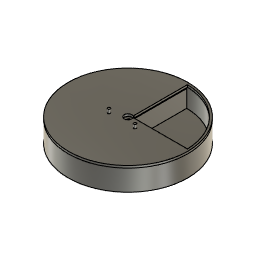
candy-dispenser (Autodesk Fusion 360 design; units mm, degrees)
Autodesk Fusion 360 part; units mm, degrees
note: some values were not read from the file. Set by a fixed rule: which sketch regions a step uses.
sketch "Floor" plane through (0, 0, 0) normal (0, 0, 1) x (1, 0, 0) in component "Container"
  circle A0 centre (0, 0) radius 80
  dimension "d25" = 160
  constraint coincident A0.centre origin
  measures "d25" diameter of A0
extrude "Extrude1" add sketch "Floor" along normal blind 3 makes body 1 in component "Container"
sketch "Walls" plane through (0, 0, 3) normal (0, 0, 1) x (-1, 0, 0) in component "Container"
  circle A0 centre (0, 0) radius 80
  circle A1 centre (0, 0) radius 77.2
  dimension "d28" = -2.8
extrude "Extrude2" add sketch "Walls" along normal blind 25 bodies 1 in component "Container"
sketch "Swiper" plane through (0, 0, 3) normal (0, 0, 1) x (-1, 0, 0) in component "Container"
  circle A0 centre (0, 0) radius 77.2
  line L0 (-80, 2.5) -> (80, 2.5)
  line L1 (80, 2.5) -> (80, -2.5)
  line L2 (80, -2.5) -> (-80, -2.5)
  line L3 (-80, -2.5) -> (-80, 2.5)
  line L4 (-80, 2.5) -> (80, -2.5) construction
  line L5 (80, 2.5) -> (-80, -2.5) construction
  line L6 (-2.5, 80) -> (2.5, 80)
  line L7 (2.5, 80) -> (2.5, -80)
  line L8 (2.5, -80) -> (-2.5, -80)
  line L9 (-2.5, -80) -> (-2.5, 80)
  line L10 (-2.5, 80) -> (2.5, -80) construction
  line L11 (2.5, 80) -> (-2.5, -80) construction
  circle A1 centre (0, 0) radius 6
  circle A2 centre (0, 0) radius 76.2
  dimension "d31" = 160
  dimension "d32" = 5
  dimension "d33" = 5
  dimension "d34" = 160
  dimension "d35" = 12
  dimension "d41" = -1
  constraint horizontal L0
  constraint perpendicular L0 L1
  constraint parallel L0 L2
  constraint parallel L1 L3
  constraint coincident L4 A0.centre
  constraint coincident L5 A0.centre
  constraint coincident A0.centre A1.centre
  constraint horizontal L6
  constraint perpendicular L6 L7
  constraint parallel L6 L8
  constraint parallel L7 L9
  constraint coincident L10 A0.centre
  constraint coincident L11 A0.centre
  measures "d31" distance of L1.end L2.end
  measures "d32" distance of L0.end L1.end
  measures "d33" distance of L7.end L8.end
  measures "d34" distance of L6.end L7.end
  measures "d35" diameter of A1
extrude "Extrude3" cut sketch "Swiper" against normal through all contours A0 L0 L7 A2 | L0 L7 A1 A2 bodies 1 in component "Container"
extrude "Extrude1'" add sketch "Swiper" along normal blind 23 separate body contours L0 L2 A1 A2 | L7 L9 A1 A2 | L0 L2 L7 A1 | L0 L7 A1 | L7 L9 A1 A2 | L2 L7 A1 | L0 L7 L9 A1 | L0 L2 L7 L9 | L2 L7 L9 A1 | L0 L2 A1 A2 | L0 L9 A1 | L0 L2 L9 A1 | L2 L9 A1 makes body 2 in component "Swiper"
sketch "Sketch1" plane through (0, 0, 26) normal (0, 0, 1) x (-1, 0, 0) in component "Swiper"
  arc A0 (2.5, -5.4544) -> (5.4544, -2.5) centre (0, 0) ccw
  line L0 (5.4544, -2.5) -> (76.159, -2.5)
  arc A1 (76.159, -2.5) -> (76.159, 2.5) centre (0, 0) ccw
  line L1 (76.159, 2.5) -> (5.4544, 2.5)
  arc A2 (5.4544, 2.5) -> (2.5, 5.4544) centre (0, 0) ccw
  line L2 (2.5, 5.4544) -> (2.5, 76.159)
  arc A3 (2.5, 76.159) -> (-2.5, 76.159) centre (0, 0) ccw
  line L3 (-2.5, 76.159) -> (-2.5, 5.4544)
  arc A4 (-2.5, 5.4544) -> (-5.4544, 2.5) centre (0, 0) ccw
  line L4 (-5.4544, 2.5) -> (-76.159, 2.5)
  arc A5 (-76.159, 2.5) -> (-76.159, -2.5) centre (0, 0) ccw
  line L5 (-76.159, -2.5) -> (-5.4544, -2.5)
  arc A6 (-5.4544, -2.5) -> (-2.5, -5.4544) centre (0, 0) ccw
  line L6 (-2.5, -5.4544) -> (-2.5, -76.159)
  arc A7 (-2.5, -76.159) -> (2.5, -76.159) centre (0, 0) ccw
  line L7 (2.5, -76.159) -> (2.5, -5.4544)
  circle A8 centre (0, 0) radius 2.5
  line L8 (-1.5, 2.5) -> (1.5, 2.5)
  line L9 (1.5, 2.5) -> (1.5, -2.5)
  line L10 (1.5, -2.5) -> (-1.5, -2.5)
  line L11 (-1.5, -2.5) -> (-1.5, 2.5)
  line L12 (-1.5, 2.5) -> (1.5, -2.5) construction
  line L13 (1.5, 2.5) -> (-1.5, -2.5) construction
  circle A9 centre (0, 0) radius 2.8
  line L14 (-1.8, -2.8) -> (-1.8, 2.8)
  line L15 (-1.8, 2.8) -> (1.8, 2.8)
  line L16 (1.8, 2.8) -> (1.8, -2.8)
  line L17 (1.8, -2.8) -> (-1.8, -2.8)
  dimension "d44" = 5
  dimension "d45" = 3
  dimension "d46" = 5
  dimension "d54" = 0.3
  dimension "d55" = -0.3
  constraint concentric A0 A8
  constraint horizontal L8
  constraint perpendicular L8 L9
  constraint parallel L8 L10
  constraint parallel L9 L11
  constraint coincident L12 A0.centre
  constraint coincident L13 A0.centre
  constraint coincident A0.centre A1.centre
  measures "d44" diameter of A8
  measures "d45" distance of L9.end L10.end
  measures "d46" distance of L8.end L9.end
extrude "Extrude3'" cut sketch "Sketch1" against normal up to surface (23 mm away) contours A8 L9 L16 | A8 L9 A9 L16 | A8 L9 A9 L16 | A8 L9 L11 | A8 L8 L9 A9 | A8 L9 L10 A9 | A8 L8 L11 A9 | L8 A9 | A8 L10 L11 A9 | L10 A9 | A8 L11 L14 | A8 L11 A9 L14 | A8 L11 A9 L14 bodies 2 in component "Swiper"
extrude "Extrude4" [suppressed] in component "Container"
extrude "Extrude1''" add 1 faces at (-53.0199, 6.1935, 0) along direction (0, 0, 1) blind 3 from surface at 28 separate body on bodies 1 makes body 3 in component "Lid"
sketch "Motor Mount" plane through (0, 0, 31) normal (0, 0, 1) x (1, 0, 0) in component "Lid"
  circle A0 centre (0, 0) radius 5
  line L0 (-17.5, 8) -> (17.5, 8) construction
  line L1 (17.5, 8) -> (17.5, -8) construction
  line L2 (17.5, -8) -> (-17.5, -8) construction
  line L3 (-17.5, -8) -> (-17.5, 8) construction
  line L4 (-17.5, 8) -> (17.5, -8) construction
  line L5 (17.5, 8) -> (-17.5, -8) construction
  circle A1 centre (17.5, 8) radius 1.75
  circle A2 centre (-17.5, 8) radius 1.75
  dimension "d58" = 10
  dimension "d62" = 35
  dimension "d63" = 16
  dimension "d64" = 3.5
  dimension "d65" = 3.5
  constraint coincident A0.centre origin
  constraint horizontal L0
  constraint perpendicular L0 L1
  constraint parallel L0 L2
  constraint parallel L1 L3
  constraint coincident L4 A0.centre
  constraint coincident L5 A0.centre
  constraint coincident L0.end L1.start
  constraint coincident L0.start L3.end
  measures "d58" diameter of A0
  measures "d62" distance of L1.end L2.end
  measures "d63" distance of L0.end L1.end
  measures "d64" diameter of A1
  measures "d65" diameter of A2
extrude "Extrude3''" add sketch "Motor Mount" along normal blind 5 contours A1 | A2 bodies 3 in component "Lid"
extrude "Extrude2'" cut sketch "Motor Mount" against normal up to surface (3 mm away) contours A0 bodies 3 in component "Lid"
component "Container" placed x (1, 0, 0) y (0, 1, 0) z (0, 0, 1) at (0, 0, 0)
component "Swiper" placed x (1, 0, 0) y (0, 1, 0) z (0, 0, 1) at (0, 0, 1)
component "Lid" placed x (-1, 0, 0) y (0, -1, 0) z (0, 0, 1) at (0, 0, 0)
named bodies: "Container", "Swiper", "Lid"
